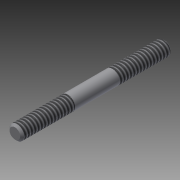
# Autodesk Inventor part: D-118538-1.422-bif
Saved by Autodesk Inventor 2014 SP2 (Build 180246200, 246)
## iProperties
Created: 2020-02-04
Part Number: D-118538-1.422-bif
Material: Generic
Catalog Web Link: www.cadenas.de
Description: BIF Tie Rod-Bimba FLAT-1
Vendor: BIMBA
Document SubType Name: Modeling
Designer: psadmin
Manufacturer: BIMBA
Mass: 0.3463 g
Surface Area: 4.10361 cm^2
Volume: 0.3463 cm^3
Density: 1 g/cm^3
Appearance: PSOLRGB-192-192-192
Category: PARTsolutions
Company: BIMBA
Title: D-118538-1.422-bif
Author: Cadenas PARTsolutions
Comments: Bimba FLAT-1
PSOL_IDENT_0: {$CADENAS_DATA\23d-libs\bimba\bimba_brand\bimba_imperial\bimba_full_line\flat_cylinders\fo1\bif_tie_
PSOL_IDENT_1: rod.prj},184 {VTYP=3D},{NB=D-118538-1.422-bif},{LINA=D-118538-1.422-bif},{NN=BIF Tie Rod},{DATE=22.0
PSOL_IDENT_2: 1.2020 09:06:04},{GEOMDATE=12.07.2017 10:25:47},{VERSION=},{LINEID=100},{WBVAR=L},{WBNUMERIC=L}  {NB=
PSOL_IDENT_3: D-118538-1.422-bif},{LINA=D-118538-1.422-bif},{KT=DUMMY},{PN=D-118538-1.422},{MODEL=D-118538},{NDM=0
PSOL_IDENT_4: .138},{L=1.42200},{HWL=0.077}
NN: BIF Tie Rod
NT: Bimba FLAT-1
NB: D-118538-1.422-bif
NBSYN: $PN.-bif
LINA: D-118538-1.422-bif
PN: D-118538-1.422
MODEL: D-118538
NDM: 0.138
L: 1.422
HWL: 0.077
SUPPLIER: BIMBA
ARTICLENO: D-118538-1.422-bif
BOMINFO: D-118538-1.422-bif
CREATOR: CADENAS GmbH
Autodesk Inventor part; units mm, degrees
ref_plane "YZ Plane" through (0, 0, 0) normal (1, 0, 0) x (0, 1, 0)
ref_plane "XZ Plane" through (0, 0, 0) normal (0, 1, 0) x (-1, 0, 0)
ref_plane "XY Plane" through (0, 0, 0) normal (0, 0, 1) x (1, 0, 0)
sketch "Sketch_3" plane through (0, 0, 0) normal (1, 0, 0) x (0, 1, 0)
  line L0 (0, -34.163) -> (0, 1.9558)
  line L1 (0, 1.9558) -> (1.2802, 1.9558)
  line L2 (1.2802, 1.9558) -> (1.7526, 1.4834)
  line L3 (1.7526, 1.4834) -> (1.7526, -33.6906)
  line L4 (1.7526, -33.6906) -> (1.2802, -34.163)
  line L5 (1.2802, -34.163) -> (0, -34.163)
  line L6 (0, -34.163) -> (0, 1.9558)
  constraints: 14 end point
revolve "Revolution1" add sketch "Sketch_3" angle 360 about axis through (0, 0, -34.163) along (0, 0, -1)
thread "Thread1" size "6-32 UNC" class "2A" standard "ANSI Unified Screw Threads" length 12.2276
thread "Thread2" size "6-32 UNC" class "2A" standard "ANSI Unified Screw Threads" length 12.2276
ref_plane "screw_XY" through (0, 0, 0) normal (0, 0, 1) x (1, 0, 0)
ref_plane "screw_YZ" through (0, 0, 0) normal (1, 0, 0) x (0, 1, 0)
ref_plane "screw_ZX" through (0, 0, 0) normal (0, 1, 0) x (0, 0, 1)
body "Solid1"
